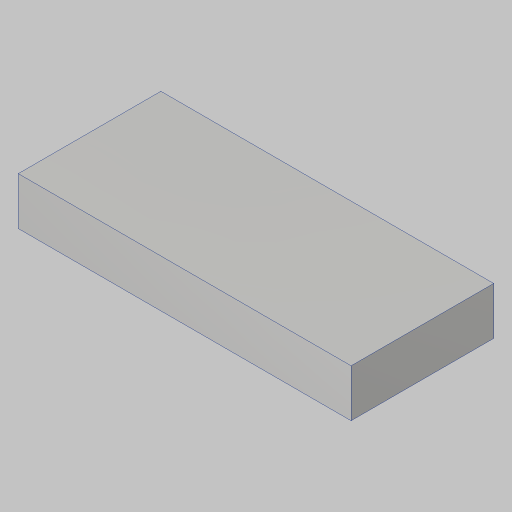
# Autodesk Inventor part: block climb
Saved by Autodesk Inventor 2023.5 (Build 275446000, 446)
## iProperties
Created: 2025-01-16
Part Number: block climb
Material: Aluminum 6061
Document SubType Name: Modeling
Designer: slick
Density: 2.7 g/cm^3
Appearance: Aluminum - Flat
Author: slick
Autodesk Inventor part; units mm, degrees
ref_plane "YZ Plane" through (0, 0, 0) normal (1, 0, 0) x (0, 1, 0)
ref_plane "XZ Plane" through (0, 0, 0) normal (0, 1, 0) x (-1, 0, 0)
ref_plane "XY Plane" through (0, 0, 0) normal (0, 0, 1) x (1, 0, 0)
sketch "Sketch1" plane through (0, 0, 0) normal (0, 1, 0) x (-1, 0, 0)
  line L0 (177.8, 76.2) -> (-177.8, 76.2)
  line L1 (-177.8, 76.2) -> (-177.8, -76.2)
  line L2 (-177.8, -76.2) -> (177.8, -76.2)
  line L3 (177.8, -76.2) -> (177.8, 76.2)
  line L4 (177.8, 76.2) -> (-177.8, -76.2) construction
  line L5 (-177.8, 76.2) -> (177.8, -76.2) construction
  point P0 (0, 0)
  dimension "d0" = 355.6
  dimension "d1" = 152.4
  constraints: 12 end point, 2 midpoint, 2 parallel, 1 horizontal, 1 perpendicular
  measures "d0" distance of L2.end L1.end
  measures "d1" distance of L1.end L0.end
extrude "Extrusion1" add sketch "Sketch1" along normal blind 50.8
body "Solid1"
